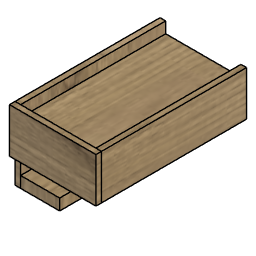
pentable (Autodesk Fusion 360 design; units mm, degrees)
description: 1 3/4 x 6 1/2 x 1/2"
description: 6 1/2 x 3 1/4 x 1/4"
description: 3 3/8 x 6 1/2 x 1/2"
description: 6 1/2 x 2 x 1/4"
description: 3 7/8 x 2 x 1/4"
Autodesk Fusion 360 part; units mm, degrees
sketch "sketch_base" plane through (0, 0, 0) normal (0, 0, 1) x (1, 0, 0)
  line L0 (0, 0) -> (44.45, 0)
  line L1 (44.45, 0) -> (44.45, 165.1)
  line L2 (44.45, 165.1) -> (0, 165.1)
  line L3 (0, 165.1) -> (0, 0)
  dimension "d1" = 44.45
  dimension "d2" = 165.1
  constraint horizontal L0
  constraint vertical L1
  constraint horizontal L2
  constraint vertical L3
  constraint coincident L0.start L3.end
  measures "d1" distance of L0.start L0.end
  measures "d2" distance of L0.start L2.end
extrude "Extrude1" add sketch "sketch_base" along normal blind 12.7 makes body 1
sketch "sketch_LSide" plane through (0, 0, 0) normal (1, 0, 0) x (0, 1, 0)
  line L0 (0, 0) -> (165.1, 0)
  line L1 (165.1, 0) -> (165.1, 82.55)
  line L2 (165.1, 82.55) -> (0, 82.55)
  line L3 (0, 82.55) -> (0, 0)
  dimension "d5" = 165.1
  dimension "d6" = 82.55
  constraint horizontal L0
  constraint vertical L1
  constraint horizontal L2
  constraint vertical L3
  constraint coincident L0.start L3.end
  measures "d5" distance of L0.start L0.end
  measures "d6" distance of L0.start L2.end
extrude "Extrude2" add sketch "sketch_LSide" against normal blind 6.35 separate body makes body 2
sketch "sketch_layers" plane through (0, 0, 0) normal (0, 1, 0) x (1, 0, 0)
  line L0 (0.0012, -6.3284) -> (0.0012, -31.7433) construction
  line L1 (44.45, -12.7) -> (44.45, -38.1) construction
  line L2 (0.0012, -31.7433) -> (85.7262, -31.7433)
  line L3 (85.7262, -31.7433) -> (85.7262, -44.4433)
  line L4 (85.7262, -44.4433) -> (0.0012, -44.4433)
  line L5 (0.0012, -44.4433) -> (0.0012, -31.7433)
  line L6 (0, 0) -> (0, -31.75) construction
  dimension "d11" = 85.725
  dimension "d12" = 12.7
  dimension "d19" = 31.75
  constraint vertical L0
  constraint vertical L1
  constraint horizontal L2
  constraint vertical L3
  constraint horizontal L4
  constraint vertical L5
  constraint coincident L6.start origin
  constraint parallel L0 L6
  measures "d11" distance of L0.end L2.end
  measures "d12" distance of L0.end L4.end
  measures "d19" distance of L6.start L6.end
extrude "Extrude3" add sketch "sketch_layers" along normal blind 165.1 separate body makes body 3
sketch "sketch_RSide" plane through (0, 0, 0) normal (0, 1, 0) x (1, 0, 0)
  line L0 (0, 0) -> (85.725, 0) construction
  line L1 (85.7264, -31.75) -> (92.0764, -31.75)
  line L2 (92.0764, -31.75) -> (92.0764, -82.55)
  line L3 (92.0764, -82.55) -> (85.7264, -82.55)
  line L4 (85.7264, -82.55) -> (85.7264, -31.75)
  dimension "d20" = 85.725
  dimension "d21" = 31.75
  constraint coincident L0.start origin
  constraint horizontal L0
  constraint horizontal L1
  constraint vertical L2
  constraint horizontal L3
  constraint vertical L4
  measures "d20" distance of L0.start L0.end
  measures "d21" distance of L0.end L1.start
extrude "Extrude4" add sketch "sketch_RSide" along normal blind 165.1 separate body makes body 4
sketch "sketch_back" plane through (0, 165.1, 0) normal (0, 1, 0) x (-1, 0, 0)
  line L0 (-0.0012, 44.4433) -> (-85.7262, 44.4433)
  line L1 (-85.7262, 44.4433) -> (-85.7262, 31.7433)
  line L2 (-85.7262, 31.7433) -> (-0.0012, 31.7433)
  line L3 (-0.0012, 31.7433) -> (-0.0012, 44.4433)
  line L4 (-92.075, 31.75, -165.1) -> (6.35, 31.75, -165.1)
  line L5 (6.35, 31.75, -165.1) -> (6.35, 82.55, -165.1)
  line L6 (6.35, 82.55, -165.1) -> (-92.075, 82.55, -165.1)
  line L7 (-92.075, 82.55, -165.1) -> (-92.075, 31.75, -165.1)
  dimension "d28" = 98.425
  dimension "d29" = 50.8
extrude "Extrude5" add sketch "sketch_back" against normal blind 6.35 separate body contours L4 L5 L6 L7 in plane through (0, 0, 0) normal (0, 1, 0) makes body 5
copy_body "Body->Comp1" bodies 1 removing the originals makes body 6 in component "Bottom"
copy_body "Body->Comp2" bodies 2 removing the originals makes body 7 in component "Right Side"
copy_body "Body->Comp3" bodies 3 removing the originals makes body 8 in component "Layer"
copy_body "Body->Comp5" bodies 4 removing the originals makes body 9 in component "Left Side"
copy_body "Body->Comp6" bodies 5 removing the originals makes body 10 in component "Back"
component "Bottom" placed x (1, 0, 0) y (0, 1, 0) z (0, 0, 1) at (0, 0, 0)
component "Right Side" placed x (1, 0, 0) y (0, 1, 0) z (0, 0, 1) at (0, 0, 0)
component "Layer" placed x (1, 0, 0) y (0, 1, 0) z (0, 0, 1) at (0, 0, 0)
component "Left Side" placed x (1, 0, 0) y (0, 1, 0) z (0, 0, 1) at (0, 0, 0)
component "Back" placed x (1, 0, 0) y (0, 1, 0) z (0, 0, 1) at (0, 0, 0)
component "Layer" placed x (1, 0, 0) y (0, 1, 0) z (0, 0, 1) at (0, 0, 0)
named bodies: "B_Bottom", "B_Layer1", "B_RSide", "B_LSide", "B_Back"
